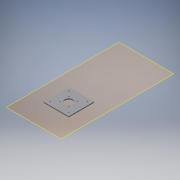
# Autodesk Inventor part: Держатель двигателя
Saved by Autodesk Inventor 2018.3 (Build 223284000, 284)
## iProperties
Created: 2018-07-22
Part Number: Держатель двигателя
Material: Типовые
Document SubType Name: Modeling
Designer: Leancher
Density: 1 g/cm^3
Appearance: По умолчанию
Author: Leancher
Autodesk Inventor part; units mm, degrees
ref_plane "YZ Plane" through (0, 0, 0) normal (1, 0, 0) x (0, 1, 0)
ref_plane "XZ Plane" through (0, 0, 0) normal (0, 1, 0) x (-1, 0, 0)
ref_plane "XY Plane" through (0, 0, 0) normal (0, 0, 1) x (1, 0, 0)
ref_plane "РабПлоскость1" through (0, 0, 0) normal (0, 0, 1) x (1, 0, 0)
sketch "Эскиз1" plane through (0, 0, 0) normal (0, 0, 1) x (1, 0, 0)
  circle A0 centre (-28.0013, -80.9009) radius 1.55
  circle A1 centre (-28.0013, -24.9009) radius 1.55
  circle A2 centre (27.9987, -24.9009) radius 1.55
  circle A3 centre (27.9987, -80.9009) radius 1.55
  line L0 (37.9987, -90.9009) -> (37.9987, -14.9009)
  line L1 (37.9987, -90.9009) -> (-38.0013, -90.9009)
  line L2 (-38.0013, -14.9009) -> (37.9987, -14.9009)
  line L3 (-38.0013, -14.9009) -> (-38.0013, -90.9009)
  circle A4 centre (-0.0013, -52.9009) radius 12
  circle A5 centre (-13.0013, -65.9009) radius 1.5
  circle A6 centre (-13.0013, -39.9009) radius 1.5
  circle A7 centre (12.9987, -39.9009) radius 1.5
  circle A8 centre (12.9987, -65.9009) radius 1.5
  point P0 (0, 0)
  dimension "d4" = 24
  constraints: 9 centre point, 8 end point, 2 horizontal, 1 vertical
  measures "d4" diameter of A4
extrude "Выдавливание1" add sketch "Эскиз1" along normal blind 3
